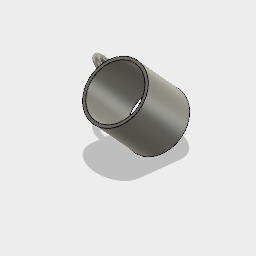
cld4 (Autodesk Fusion 360 design; units mm, degrees)
Autodesk Fusion 360 part; units mm, degrees
cylinder "圆柱体基本要素1" add diameter 20 height 20 placed x (1, 0, 0) y (0, 0, -1) z (0, 1, 0) at (0, 0, 0) makes body 1
cylinder "圆柱体基本要素2" add diameter 18 height 20 placed x (1, 0, 0) y (0, 0, -1) z (0, 1, 0) at (28.2708, 0, -1.1926) separate body makes body 2
torus "圆环体基本要素1" add centre line diameter 12 section diameter 2 placed x (1, 0, 0) y (0, 0, -1) z (0, 1, 0) at (59.0183, 0, 0.6928) separate body makes body 3
move_body "MoveFace1" bodies 3 to x (0.173648, -0.984808, 0) y (0, 0, 1) z (-0.984808, -0.173648, 0) at (-41.568, 64.9025, 0.6928) on bodies 3
move_body "MoveFace2" bodies 3 to x (1, 0, 0) y (0, 1, 0) z (0, 0, 1) at (20, 5, 0) on bodies 3
combine "合并1" operation add target body 3 tool bodies 1
move_body "移动1" bodies 3 to x (1, 0, 0) y (0, 1, 0) z (0, 0, 1) at (90, 25, 0)
move_body "移动2" bodies 3 to x (0.173648, -0.984808, 0) y (0.984808, 0.173648, 0) z (0, 0, 1) at (34.0492, 90.5783, 0)
move_body "对齐1" bodies 2 to x (-0.173648, 0.984808, 0) y (-0.984808, -0.173648, 0) z (0, 0, 1) at (98.9031, -18.0816, 1.1926)
ref_plane "工作平面1" through (92.0243, 9.4125, 0) normal (0.984808, 0.173648, 0) x (0.173648, -0.984808, 0)
move_body "移动3" bodies 3 2 to x (0.074716, 0.694272, 0.715824) y (-0.920712, 0.323744, -0.217895) z (-0.383022, -0.642788, 0.663414) at (70.5155, -44.0494, -74.1892)
combine "合并2" operation cut target body 3 tool bodies 2
